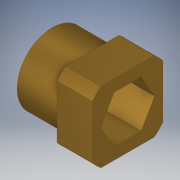
# Autodesk Inventor part: T81H-RS81
Saved by Autodesk Inventor 2017.1 (Build 211199000, 199)
## iProperties
Category: Loose
Company: Autodesk Inc.
Created: 2016-12-26
Part Number: T81H-RS81
Material: Aluminum 6061
Document SubType Name: Modeling
Designer: Autodesk Inc.
Density: 2.7 g/cm^3
Appearance: Brass - Satin
Catalog Web Link: www.banebots.com
Vendor: BaneBots
Author: Autodesk Inc.
Keywords: Gray Tote
Autodesk Inventor part; units mm, degrees
ref_plane "YZ Plane" through (0, 0, 0) normal (1, 0, 0) x (0, 1, 0)
ref_plane "XZ Plane" through (0, 0, 0) normal (0, 1, 0) x (-1, 0, 0)
ref_plane "XY Plane" through (0, 0, 0) normal (0, 0, 1) x (1, 0, 0)
sketch "Sketch1" plane through (0, 0, 0) normal (0, 1, 0) x (-1, 0, 0)
  line L0 (6.35, -3.6662) -> (0, -7.3323)
  line L1 (0, -7.3323) -> (-6.35, -3.6662)
  line L2 (-6.35, -3.6662) -> (-6.35, 3.6662)
  line L3 (-6.35, 3.6662) -> (0, 7.3323)
  line L4 (0, 7.3323) -> (6.35, 3.6662)
  line L5 (6.35, 3.6662) -> (6.35, -3.6662)
  line L6 (9.525, 7.1772) -> (9.525, -7.1772)
  line L7 (-9.525, 7.1772) -> (-9.525, -7.1772)
  line L8 (7.1772, 9.525) -> (-7.1772, 9.525)
  line L9 (7.1772, -9.525) -> (-7.1772, -9.525)
  arc A0 (7.1772, -9.525) -> (9.525, -7.1772) centre (0, 0) ccw
  arc A1 (9.525, 7.1772) -> (7.1772, 9.525) centre (0, 0) ccw
  arc A2 (-7.1772, 9.525) -> (-9.525, 7.1772) centre (0, 0) ccw
  arc A3 (-9.525, -7.1772) -> (-7.1772, -9.525) centre (0, 0) ccw
  dimension "d0" = 12.7
  dimension "d9" = 9.525
  dimension "d10" = 9.525
  dimension "d11" = 9.525
  dimension "d12" = 9.525
  constraints: 20 end point, 8 point on circle, 4 centre point, 3 vertical, 2 coincident, 2 horizontal, 13 other
  measures "d0" distance between parallel lines of L2 L5
  measures "d9" distance from line of point (0, 0) L6
  measures "d10" distance from line of L7 point (0, 0)
  measures "d11" distance from line of L8 point (0, 0)
  measures "d12" distance from line of L9 point (0, 0)
extrude "Extrusion1" add sketch "Sketch1" against normal blind 9.525 contours L0 L1 L2 L3 L4 L5 | L6 A0 L9 A3 L7 A2 L8 A1
sketch "Sketch2" plane through (0, -9.525, 0) normal (0, -1, 0) x (0.7071, 0, 0.7071)
  circle A0 centre (0, 0) radius 9.525
  dimension "d4" = 19.05
  constraints: 1 centre point, 1 coincident
  measures "d4" diameter of A0
extrude "Extrusion2" add sketch "Sketch2" along normal blind 10.795
extrude "Extrusion3" cut sketch "Sketch1" against normal through all contours L0 L1 L2 L3 L4 L5
equation "\"d10\" = d9"
equation "\"d11\" = d9"
equation "\"d12\" = d11"
body "Solid1"
